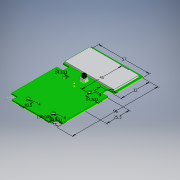
# Autodesk Inventor part: Cheapstat
Saved by Autodesk Inventor 2016 (Build 200138000, 138)
## iProperties
Created: 2015-05-13
Part Number: Cheapstat
Material: Generic
Document SubType Name: Modeling
Designer: David
Density: 1 g/cm^3
Appearance: Dark Green
Mass: 12.0181 g
Surface Area: 117.683 cm^2
Volume: 12.0181 cm^3
Author: David
Autodesk Inventor part; units mm, degrees
ref_plane "YZ Plane" through (0, 0, 0) normal (1, 0, 0) x (0, 1, 0)
ref_plane "XZ Plane" through (0, 0, 0) normal (0, 1, 0) x (-1, 0, 0)
ref_plane "XY Plane" through (0, 0, 0) normal (0, 0, 1) x (1, 0, 0)
sketch "Sketch1" plane through (0, 0, 0) normal (0, 1, 0) x (-1, 0, 0)
  line L0 (-28.5, -48) -> (28.5, -48)
  line L1 (28.5, 48) -> (-28.5, -48) construction
  line L2 (-28.5, 48) -> (28.5, -48) construction
  line L3 (-28.5, -48) -> (-28.5, -16)
  line L4 (-28.5, -16) -> (-21.5, -16)
  line L5 (-21.5, -16) -> (-21.5, -9)
  line L6 (-21.5, -9) -> (-28.5, -9)
  line L7 (0, -48) -> (0, 48)
  line L8 (21.5, -16) -> (21.5, -9)
  line L9 (28.5, -16) -> (21.5, -16)
  line L10 (21.5, -9) -> (28.5, -9)
  line L11 (-28.5, -9) -> (-28.5, 16.5)
  line L12 (-28.5, 16.5) -> (28.5, 16.5)
  line L13 (21.5, 42) -> (28.5, 42)
  line L14 (-28.5, -48) -> (-13.5, -48)
  line L15 (-13.5, -48) -> (-13.5, -3)
  line L16 (28.5, 42) -> (28.5, -9)
  line L17 (28.5, -16) -> (28.5, -48)
  line L18 (-28.5, 16.5) -> (-28.5, 42)
  line L19 (-28.5, -3) -> (-13.967, -3)
  circle A0 centre (-13.967, -3) radius 2
  line L20 (-28.5, 37) -> (-13.967, 37)
  circle A1 centre (13.967, -3) radius 2
  line L21 (21.5, 48) -> (21.5, 42)
  line L22 (-28.5, 42) -> (-21.5, 42)
  line L23 (-21.5, 42) -> (-21.5, 48)
  line L24 (-21.5, 48) -> (21.5, 48)
  line L25 (-13.967, 48) -> (-13.967, 37.5)
  line L26 (-13.967, 48) -> (-3.467, 48) construction
  line L27 (13.967, 48) -> (13.967, 37.5)
  circle A2 centre (13.967, 37.5) radius 2
  circle A3 centre (-13.967, 37.5) radius 2
  point P0 (0, 0)
  dimension "d0" = 57
  dimension "d1" = 96
  dimension "d2" = 32
  dimension "d3" = 7
  dimension "d4" = 7
  dimension "d5" = 25.5
  dimension "d7" = 45
  dimension "d40" = 14.533
  dimension "d41" = 4
  dimension "d42" = 14.533
  dimension "d50" = 14.533
  dimension "d57" = 7
  dimension "d59" = 10.5
  dimension "d60" = 90
  dimension "d61" = 10.5
  dimension "d62" = 4
  dimension "d63" = 4
  constraints: 56 end point, 8 perpendicular, 5 symmetric about line, 5 vertical, 4 centre point, 4 point on line, 3 coincident, 3 horizontal, 3 midpoint, 1 collinear, 1 other
  measures "d0" distance of L0.end L0.start
  measures "d1" distance of L0.start L2.start
  measures "d2" distance of L0.start L3.end
  measures "d3" distance of L3.end L4.end
  measures "d4" distance of L4.end L5.end
  measures "d5" distance of L6.end L11.end
  measures "d7" distance of L15.end L14.end
  measures "d40" distance of L19.start L19.end
  measures "d41" diameter of A0
  measures "d42" distance of L20.start L20.end
  measures "d50" distance from line of A1.centre L16
  measures "d57" distance of L18.end L22.end
  measures "d59" distance of L25.start L25.end
  measures "d60" angle of L25 L26
  measures "d61" distance of L27.start L27.end
  measures "d62" diameter of A2
  measures "d63" diameter of A3
extrude "Extrusion2" add sketch "Sketch1" along normal blind 1.6 contours L3 L4 L5 L6 L11 L19 A0 L15 L0 | L15 A0 L19 L11 L12 L7 L0 | L7 L12 L16 L10 L8 L9 L17 L0 | A0 | L12 L18 L20 A3 L25 L24 L7 | L7 L24 L21 L13 L16 L12 | L25 A3 L20 L18 L22 L23 L24 | A3 | A1 | A2
sketch "Sketch3" plane through (0, 1.6, 0) normal (0, 1, 0) x (1, 0, 0)
  line L0 (28.5, 48) -> (-28.5, 48) projected
  line L1 (28.5, 48) -> (27.5, 48)
  line L2 (27.5, 48) -> (27.5, 45)
  line L3 (27.5, 45) -> (28.5, 45)
  line L4 (28.5, 45) -> (28.5, 48)
  line L5 (27.5, 45) -> (-27.5, 45)
  line L6 (-27.5, 45) -> (-27.5, 17)
  line L7 (-27.5, 17) -> (27.5, 17)
  line L8 (27.5, 17) -> (27.5, 45)
  point P0 (0, 0)
  dimension "d16" = 1
  dimension "d17" = 3
  dimension "d18" = 55
  dimension "d19" = 28
  constraints: 16 end point, 4 parallel, 2 horizontal, 2 perpendicular
  measures "d16" distance of L3.end L2.end
  measures "d17" distance of L2.end L1.end
  measures "d18" distance of L7.end L6.end
  measures "d19" distance of L6.end L5.end
extrude "Extrusion3" add sketch "Sketch3" along normal blind 2 contours L8 L7 L6 L5
sketch "Sketch4" plane through (0, 1.6, 0) normal (0, 1, 0) x (1, 0, 0)
  line L0 (-2.5, 8.5) -> (2.5, 8.5)
  line L1 (2.5, 8.5) -> (2.5, 13.5)
  line L2 (2.5, 13.5) -> (-2.5, 13.5)
  line L3 (-2.5, 13.5) -> (-2.5, 8.5)
  line L4 (-2.5, 8.5) -> (2.5, 13.5) construction
  line L5 (2.5, 8.5) -> (-2.5, 13.5) construction
  point P0 (0, 0)
  point P1 (-21.5, -46.725)
  point P2 (21.5, -46.725)
  constraints: 12 end point, 2 parallel, 1 horizontal, 1 perpendicular
extrude "Extrusion4" add sketch "Sketch4" along normal blind 3
sketch "Sketch5" plane through (0, 4.6, 0) normal (0, 1, 0) x (1, 0, 0)
  point P0 (0, 0)
sketch "Sketch6" plane through (0, 4.6, 0) normal (0, 1, 0) x (1, 0, 0)
  line L0 (2.5, 8.5) -> (2.5, 13.5) projected
  line L1 (2.5, 13.5) -> (0, 13.5)
  line L2 (0, 13.5) -> (0, 11)
  line L3 (0, 11) -> (2.5, 11)
  line L4 (2.5, 11) -> (2.5, 13.5)
  line L5 (-1.5, 9.5) -> (1.5, 9.5)
  line L6 (1.5, 9.5) -> (1.5, 12.5)
  line L7 (1.5, 12.5) -> (-1.5, 12.5)
  line L8 (-1.5, 12.5) -> (-1.5, 9.5)
  line L9 (-1.5, 9.5) -> (1.5, 12.5) construction
  line L10 (1.5, 9.5) -> (-1.5, 12.5) construction
  point P0 (0, 0)
  dimension "d29" = 3
  dimension "d30" = 3
  constraints: 20 end point, 4 parallel, 2 horizontal, 2 midpoint, 2 perpendicular
  measures "d29" distance of L7.end L6.end
  measures "d30" distance of L6.end L5.end
extrude "Extrusion5" add sketch "Sketch6" along normal blind 3.5 contours L6 L5 L8 L7 L2 L3 | L3 L2 L7 L6
sketch "Sketch7" plane through (0, 0, 0) normal (0, -1, 0) x (1, 0, 0)
  line L0 (28.5, -48) -> (-28.5, -48) projected
  line L1 (-28.5, -48) -> (-26.5, -48)
  line L2 (-26.5, -48) -> (-26.5, -5)
  line L3 (-26.5, -5) -> (-28.5, -5)
  line L4 (-28.5, -5) -> (-28.5, -48)
  line L5 (-26.5, -5) -> (-18.5, -5)
  line L6 (-18.5, -5) -> (-18.5, 2)
  line L7 (-18.5, 2) -> (-26.5, 2)
  line L8 (-26.5, 2) -> (-26.5, -5)
  line L9 (-26.5, 2) -> (-26.5, 17)
  line L10 (-26.5, 17) -> (0, 17)
  line L11 (-18.5, 32) -> (-26.5, 32)
  line L12 (-18.5, 39) -> (-18.5, 32)
  line L13 (-26.5, 39) -> (-18.5, 39)
  line L14 (-26.5, 32) -> (-26.5, 39)
  point P0 (0, 0)
  dimension "d33" = 2
  dimension "d34" = 43
  dimension "d35" = 8
  dimension "d36" = 7
  dimension "d37" = 15
  constraints: 28 end point, 4 parallel, 4 symmetric about line, 3 perpendicular, 2 horizontal, 1 vertical
  measures "d33" distance of L3.end L2.end
  measures "d34" distance of L2.end L1.end
  measures "d35" distance of L7.end L6.end
  measures "d36" distance of L6.end L5.end
  measures "d37" distance of L7.end L9.end
extrude "Extrusion6" add sketch "Sketch7" along normal blind 4 contours L8 L7 L6 L5 | L11 L14 L13 L12
extrude "Extrusion7" cut sketch "Sketch1" along normal blind 10 contours A0
extrude "Extrusion8" cut sketch "Sketch1" along normal blind 10 contours A1
extrude "Extrusion9" cut sketch "Sketch1" along normal blind 10 contours A3 | A2
body "Solid2"
